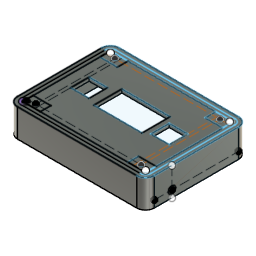
scamp-oled-case v5 (Autodesk Fusion 360 design; units mm, degrees)
Autodesk Fusion 360 part; units mm, degrees
note: some values were not read from the file. Set by a fixed rule: which sketch regions a step uses.
sketch "Sketch1" plane through (0, 0, 0) normal (0, 0, 1) x (1, 0, 0)
  line L0 (1, 0) -> (69, 0)
  line L1 (70, 1) -> (70, 49)
  line L2 (69, 50) -> (1, 50)
  line L3 (0, 49) -> (0, 1)
  line L4 (0, 2.5) -> (70, 2.5) construction
  line L5 (0, 47.5) -> (70, 47.5) construction
  line L6 (65, 50) -> (65, 0) construction
  line L7 (5, 50) -> (5, 0) construction
  line L8 (0, 50) -> (10, 50)
  line L9 (10, 50) -> (10, 44)
  line L10 (10, 44) -> (0, 44)
  line L11 (0, 44) -> (0, 50)
  line L12 (70, 50) -> (60, 50)
  line L13 (60, 50) -> (60, 44)
  line L14 (60, 44) -> (70, 44)
  line L15 (70, 44) -> (70, 50)
  line L16 (0, 0) -> (10, 0)
  line L17 (10, 0) -> (10, 6)
  line L18 (10, 6) -> (0, 6)
  line L19 (0, 6) -> (0, 0)
  line L20 (70, 0) -> (60, 0)
  line L21 (60, 0) -> (60, 6)
  line L22 (60, 6) -> (70, 6)
  line L23 (70, 6) -> (70, 0)
  line L24 (6.8, 50) -> (6.8, 0) construction
  line L25 (63, 0) -> (63, 50) construction
  line L26 (63, 31) -> (52.5, 31)
  line L27 (52.5, 31) -> (52.5, 20.5)
  line L28 (52.5, 20.5) -> (63, 20.5)
  line L29 (63, 20.5) -> (63, 31)
  line L30 (6.8, 31) -> (17.3, 31)
  line L31 (17.3, 31) -> (17.3, 20.5)
  line L32 (17.3, 20.5) -> (6.8, 20.5)
  line L33 (6.8, 20.5) -> (6.8, 31)
  line L34 (22, 34.5) -> (49.5, 34.5)
  line L35 (49.5, 34.5) -> (49.5, 18.5)
  line L36 (49.5, 18.5) -> (22, 18.5)
  line L37 (22, 18.5) -> (22, 34.5)
  circle A0 centre (5, 47.5) radius 1
  circle A1 centre (65, 47.5) radius 1
  circle A2 centre (5, 2.5) radius 1
  circle A3 centre (65, 2.5) radius 1
  arc A4 (1, 50) -> (0, 49) centre (1, 49) ccw
  arc A5 (70, 49) -> (69, 50) centre (69, 49) ccw
  arc A6 (0, 1) -> (1, 0) centre (1, 1) ccw
  arc A7 (69, 0) -> (70, 1) centre (69, 1) ccw
  line L38 (72, 1) -> (72, 49)
  arc A8 (72, 49) -> (69, 52) centre (69, 49) ccw
  line L39 (69, 52) -> (1, 52)
  arc A9 (1, 52) -> (-2, 49) centre (1, 49) ccw
  line L40 (-2, 49) -> (-2, 1)
  arc A10 (-2, 1) -> (1, -2) centre (1, 1) ccw
  line L41 (1, -2) -> (69, -2)
  arc A11 (69, -2) -> (72, 1) centre (69, 1) ccw
  line L42 (1, -4) -> (69, -4)
  arc A12 (69, -4) -> (74, 1) centre (69, 1) ccw
  line L43 (74, 1) -> (74, 49)
  arc A13 (74, 49) -> (69, 54) centre (69, 49) ccw
  line L44 (69, 54) -> (1, 54)
  arc A14 (1, 54) -> (-4, 49) centre (1, 49) ccw
  line L45 (-4, 49) -> (-4, 1)
  arc A15 (-4, 1) -> (1, -4) centre (1, 1) ccw
  dimension "d1" = 2
  dimension "d2" = 4
  dimension "d3" = 5
  dimension "d4" = 5
  dimension "d5" = 2.5
  dimension "d6" = 2.5
  dimension "d7" = 10
  dimension "d8" = 6
  dimension "d9" = 10
  dimension "d10" = 6
  dimension "d11" = 10
  dimension "d12" = 6
  dimension "d13" = 10
  dimension "d14" = 6
  dimension "d15" = 6.8
  dimension "d16" = 7
  dimension "d17" = 10.5
  dimension "d18" = 10.5
  dimension "d19" = 10.5
  dimension "d20" = 10.5
  dimension "d21" = 19
  dimension "d22" = 19
  dimension "d23" = 27.5
  dimension "d24" = 16
  dimension "d25" = 22
  dimension "d34" = 2
  dimension "d35" = 2
  dimension "d36" = 2
  dimension "d37" = 2
  dimension "d41" = 1
  dimension "d42" = 1
  dimension "d43" = 1
  dimension "d44" = 1
  dimension "d45" = 15.5
  constraint horizontal L0
  constraint vertical L1
  constraint horizontal L2
  constraint vertical L3
  constraint coincident L16.start L19.end
  constraint coincident L3 L4.start
  constraint perpendicular L3 L4
  constraint coincident L1 L4.end
  constraint coincident L3 L5.start
  constraint perpendicular L3 L5
  constraint coincident L1 L5.end
  constraint coincident L2 L6.start
  constraint perpendicular L2 L6
  constraint coincident L0 L6.end
  constraint coincident L2 L7.start
  constraint perpendicular L2 L7
  constraint coincident L0 L7.end
  constraint horizontal L8
  constraint vertical L9
  constraint horizontal L10
  constraint vertical L11
  constraint horizontal L12
  constraint vertical L13
  constraint horizontal L14
  constraint vertical L15
  constraint horizontal L16
  constraint vertical L17
  constraint horizontal L18
  constraint vertical L19
  constraint horizontal L20
  constraint vertical L21
  constraint horizontal L22
  constraint vertical L23
  constraint coincident L2 L24.start
  constraint coincident L0 L24.end
  constraint perpendicular L0 L24
  constraint coincident L20 L25.start
  constraint coincident L2 L25.end
  constraint perpendicular L2 L25
  constraint horizontal L26
  constraint vertical L27
  constraint horizontal L28
  constraint vertical L29
  constraint coincident L25 L26.start
  constraint horizontal L30
  constraint vertical L31
  constraint horizontal L32
  constraint vertical L33
  constraint coincident L24 L30.start
  constraint horizontal L34
  constraint vertical L35
  constraint horizontal L36
  constraint vertical L37
  constraint coincident L7 A0.centre
  constraint coincident L5 A0.centre
  constraint coincident L6 A1.centre
  constraint coincident L5 A1.centre
  constraint coincident L7 A2.centre
  constraint coincident L4 A2.centre
  constraint coincident L6 A3.centre
  constraint coincident L4 A3.centre
  constraint coincident L8.start L3
  constraint coincident L8.start L2
  constraint tangent L3 A4
  constraint tangent L2 A4
  constraint coincident L12.start L2
  constraint coincident L12.start L1
  constraint tangent L2 A5
  constraint tangent L1 A5
  constraint coincident L16.start L3
  constraint coincident L16.start L0
  constraint tangent L3 A6
  constraint tangent L0 A6
  constraint coincident L20.start L1
  constraint coincident L20.start L0
  constraint tangent L1 A7
  constraint tangent L0 A7
  measures "d3" distance of L3 L7
  measures "d4" distance of L1 L6
  measures "d5" distance of L2 L5
  measures "d6" distance of L0 L4
  measures "d7" distance of L8.start L8.end
  measures "d8" distance of L8.start L10.end
  measures "d9" distance of L12.start L12.end
  measures "d10" distance of L12.start L14.end
  measures "d11" distance of L16.start L16.end
  measures "d12" distance of L16.start L18.end
  measures "d13" distance of L20.start L20.end
  measures "d14" distance of L20.start L22.end
  measures "d15" distance of L3 L24
  measures "d16" distance of L1 L25
  measures "d17" distance of L26.start L26.end
  measures "d18" distance of L26.start L28.end
  measures "d19" distance of L30.start L30.end
  measures "d20" distance of L30.start L32.end
  measures "d21" distance of L2 L26
  measures "d22" distance of L2 L30
  measures "d23" distance of L34.start L34.end
  measures "d24" distance of L34.start L36.end
  measures "d25" distance of L3 L37
  measures "d34" diameter of A0
  measures "d35" diameter of A1
  measures "d36" diameter of A2
  measures "d37" diameter of A3
  measures "d41" radius of A4
  measures "d42" radius of A5
  measures "d43" radius of A6
  measures "d44" radius of A7
  measures "d45" distance of L2 L34
extrude "Extrude1" add sketch "Sketch1" against normal blind 16 contours L42 A12 L43 A13 L44 A14 L45 A15 makes body 1
extrude "Extrude2" add sketch "Sketch1" against normal blind 2 contours L38 A8 L39 A9 L40 A10 L41 A11 bodies 1
extrude "Extrude3" add sketch "Sketch1" against normal blind 7 contours L0 L3 L16 L17 L18 L19 A6 | L16 L19 A6 | L0 L1 L20 L21 L22 L23 A7 | L20 L23 A7 | L2 L3 L8 L9 L10 L11 A4 | L8 L11 A4 | L1 L2 L12 L13 L14 L15 A5 | L12 L15 A5 | A0 | A1 | A2 | A3 bodies 1
extrude "Extrude4" add sketch "Sketch1" against normal blind 2 separate body contours L0 L1 L2 L3 L9 L10 L13 L14 L17 L18 L21 L22 makes body 2
extrude "Extrude5" cut sketch "Sketch1" against normal blind 12 from surface at -2 contours A0 | A1 | A2 | A3 bodies 1
sketch "Sketch2" plane through (74, 0, 0) normal (1, 0, 0) x (0, 1, 0)
  line L0 (49, 0) -> (1, 0)
  line L1 (1, 0) -> (1, -16)
  line L2 (1, -16) -> (49, -16)
  line L3 (49, -16) -> (49, 0)
  line L4 (11, 0) -> (11, -16) construction
  line L5 (1, -12) -> (49, -12) construction
  circle A0 centre (11, -12) radius 2
  dimension "d47" = 4
  dimension "d50" = 10
  dimension "d51" = 4
  constraint coincident L1 L5.start
  constraint perpendicular L1 L5
  constraint coincident L3 L5.end
  constraint coincident L5 A0.centre
  constraint coincident L4 A0.centre
  measures "d47" distance of L2 L5
  measures "d50" distance of L1 L4
  measures "d51" diameter of A0
extrude "Extrude7" cut sketch "Sketch2" against normal blind 6 contours A0 bodies 1
